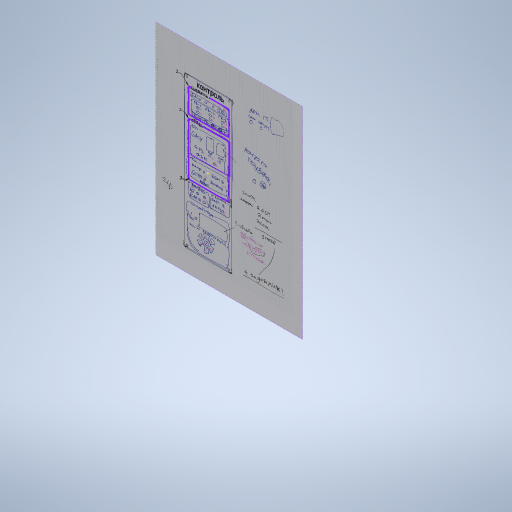
# Autodesk Inventor part: блок контроля
Saved by Autodesk Inventor 2023.1 (Build 271208000, 208)
## iProperties
Created: 2023-02-23
Part Number: блок контроля
Material: Типовые
Document SubType Name: Modeling
Designer: User
Density: 1 g/cm^3
Appearance: По умолчанию
Author: User
Autodesk Inventor part; units mm, degrees
ref_plane "YZ Plane" through (0, 0, 0) normal (1, 0, 0) x (0, 1, 0)
ref_plane "XZ Plane" through (0, 0, 0) normal (0, 1, 0) x (-1, 0, 0)
ref_plane "XY Plane" through (0, 0, 0) normal (0, 0, 1) x (1, 0, 0)
sketch "Эскиз1" plane through (0, 0, 0) normal (0, 0, 1) x (1, 0, 0)
  line L0 (-35, 111.5) -> (35, 111.5)
  line L1 (35, 111.5) -> (35, -111.5)
  line L2 (35, -111.5) -> (-35, -111.5)
  line L3 (-35, -111.5) -> (-35, 111.5)
  line L4 (0, -156.1) -> (0, 156.1) projected
  line L5 (-49, 0) -> (49, 0) projected
  line L6 (-30, 106.5) -> (30, 106.5)
  line L7 (30, 106.5) -> (30, -106.5)
  line L8 (30, -106.5) -> (-30, -106.5)
  line L9 (-30, -106.5) -> (-30, 106.5)
  circle A0 centre (-31, 107.5) radius 1.5
  circle A1 centre (-31, 107.5) radius 3.5
  circle A2 centre (31, 107.5) radius 1.5
  circle A3 centre (31, 107.5) radius 3.5
  circle A4 centre (-31, -107.5) radius 1.5
  circle A5 centre (-31, -107.5) radius 3.5
  circle A6 centre (31, -107.5) radius 1.5
  circle A7 centre (31, -107.5) radius 3.5
  point P0 (0, 0)
  dimension "d0" = 70
  dimension "d1" = 223
  dimension "d2" = 5
  dimension "d3" = 5
  dimension "d4" = 5
  dimension "d5" = 5
  dimension "d6" = 3
  dimension "d7" = 7
  dimension "d8" = 3
  dimension "d9" = 7
  dimension "d10" = 3
  dimension "d11" = 7
  dimension "d12" = 3
  dimension "d13" = 7
  dimension "d14" = 1
  dimension "d15" = 1
  dimension "d16" = 1
  dimension "d17" = 1
  dimension "d18" = 1
  dimension "d19" = 1
  dimension "d20" = 1
  dimension "d21" = 1
  constraints: 16 end point, 8 centre point, 4 coincident, 4 parallel, 2 horizontal, 2 perpendicular, 2 other
  measures "d0" distance between parallel lines of L1 L3
  measures "d1" distance between parallel lines of L2 L0
  measures "d2" distance between parallel lines of L6 L0
  measures "d3" distance between parallel lines of L1 L7
  measures "d4" distance between parallel lines of L3 L9
  measures "d5" distance between parallel lines of L2 L8
  measures "d6" diameter of A0
  measures "d7" diameter of A1
  measures "d8" diameter of A2
  measures "d9" diameter of A3
  measures "d10" diameter of A4
  measures "d11" diameter of A5
  measures "d12" diameter of A6
  measures "d13" diameter of A7
  measures "d14" distance from line of L9 A0.centre
  measures "d15" distance from line of A0.centre L6
  measures "d16" distance from line of L8 A4.centre
  measures "d17" distance from line of L9 A4.centre
  measures "d18" distance from line of L8 A6.centre
  measures "d19" distance from line of A7.centre L7
  measures "d20" distance from line of L6 A2.centre
  measures "d21" distance from line of L7 A2.centre
extrude "Выдавливание1" add sketch "Эскиз1" along normal blind 2 contours L0 L4 L6 A1 L9 L5 L3 | L0 L1 L5 L7 A3 L6 L4 | L5 L9 A5 L8 L4 L2 L3 | L6 A3 L7 L5 L4 | L4 L5 L9 A1 L6 | L5 L4 L8 A5 L9 | L1 L2 L4 L8 A7 L7 L5 | L5 L7 A7 L8 L4 | A1 L9 A0 L6 | L6 A0 L9 A1 | A3 L7 A2 L6 | L6 A2 L7 A3 | A5 L8 A4 L9 | L9 A4 L8 A5 | A7 L8 A6 L7 | L7 A6 L8 A7
fillet "Сопряжение1" radius 3 4 edges at (-35, -111.5, 1) (-35, 111.5, 1) (35, 111.5, 1) (35, -111.5, 1)
sketch "Эскиз2" plane through (0, 0, 2) normal (0, 0, 1) x (1, 0, 0)
  line L0 (-76.7343, 154.5381) -> (139.2503, 154.5381) construction
  line L1 (139.2503, 154.5381) -> (139.2503, -142.4726) construction
  line L2 (139.2503, -142.4726) -> (-76.7343, -142.4726) construction
  line L3 (-76.7343, -142.4726) -> (-76.7343, 154.5381) construction
  line L4 (-16.9113, 107.032) -> (17.9169, 107.032) construction
  line L5 (17.9169, 107.032) -> (17.9169, 100.7451) construction
  line L6 (17.9169, 100.7451) -> (-16.9113, 100.7451) construction
  line L7 (-16.9113, 100.7451) -> (-16.9113, 107.032) construction
  line L8 (31.258, 95.6248) -> (31.258, 62.5304)
  line L9 (29.258, 60.5304) -> (-27.4022, 60.5304)
  line L10 (-29.4022, 62.5304) -> (-29.4022, 95.6248)
  arc A0 (-27.4022, 97.6248) -> (-29.4022, 95.6248) centre (-27.4022, 95.6248) ccw
  arc A1 (31.258, 95.6248) -> (29.258, 97.6248) centre (29.258, 95.6248) ccw
  arc A2 (29.258, 60.5304) -> (31.258, 62.5304) centre (29.258, 62.5304) ccw
  arc A3 (-29.4022, 62.5304) -> (-27.4022, 60.5304) centre (-27.4022, 62.5304) ccw
  arc A4 (-27.4022, 96.6248) -> (-28.4022, 95.6248) centre (-27.4022, 95.6248) ccw
  line L11 (-28.4022, 95.6248) -> (-28.4022, 62.5304)
  arc A5 (-28.4022, 62.5304) -> (-27.4022, 61.5304) centre (-27.4022, 62.5304) ccw
  line L12 (-27.4022, 61.5304) -> (29.258, 61.5304)
  arc A6 (29.258, 61.5304) -> (30.258, 62.5304) centre (29.258, 62.5304) ccw
  line L13 (30.258, 62.5304) -> (30.258, 95.6248)
  arc A7 (30.258, 95.6248) -> (29.258, 96.6248) centre (29.258, 95.6248) ccw
  line L14 (-25.7338, 97.6248) -> (-25.7338, 96.6248)
  line L15 (-24.8875, 98.8096) -> (-4.5511, 98.8096) construction
  line L16 (-4.5511, 98.8096) -> (-4.5511, 95.9853) construction
  line L17 (-4.5511, 95.9853) -> (-24.8875, 95.9853) construction
  line L18 (-24.8875, 95.9853) -> (-24.8875, 98.8096) construction
  line L19 (1.4856, 96.6248) -> (1.4856, 97.6248)
  line L20 (-27.4022, 97.6248) -> (-25.7338, 97.6248)
  line L21 (1.4856, 97.6248) -> (29.258, 97.6248)
  line L22 (29.258, 96.6248) -> (1.4856, 96.6248)
  line L23 (-25.7338, 96.6248) -> (-27.4022, 96.6248)
  line L24 (31.258, 54.2392) -> (31.258, 12.1954)
  line L25 (-29.4022, 12.1954) -> (-29.4022, 54.2392)
  arc A8 (-27.4022, 56.2392) -> (-29.4022, 54.2392) centre (-27.4022, 54.2392) ccw
  arc A9 (31.258, 54.2392) -> (29.258, 56.2392) centre (29.258, 54.2392) ccw
  arc A10 (-27.4022, 55.2392) -> (-28.4022, 54.2392) centre (-27.4022, 54.2392) ccw
  line L26 (-28.4022, 54.2392) -> (-28.4022, 12.1954)
  line L27 (30.258, 12.1954) -> (30.258, 54.2392)
  arc A11 (30.258, 54.2392) -> (29.258, 55.2392) centre (29.258, 54.2392) ccw
  line L28 (-25.7338, 56.2392) -> (-25.7338, 55.2392)
  line L29 (-24.6363, 58.99) -> (-4.7949, 58.99) construction
  line L30 (-4.7949, 58.99) -> (-4.7949, 51.439) construction
  line L31 (-4.7949, 51.439) -> (-24.6363, 51.439) construction
  line L32 (-24.6363, 51.439) -> (-24.6363, 58.99) construction
  line L33 (31.258, 12.1954) -> (31.258, -20.0847)
  line L34 (29.258, -22.0847) -> (-27.4022, -22.0847)
  line L35 (-29.4022, -20.0847) -> (-29.4022, 12.1954)
  line L36 (29.9651, 12.1954) -> (29.9651, -20.0847)
  line L37 (28.9651, -21.0847) -> (-27.4022, -21.0847)
  line L38 (-28.4022, -20.0847) -> (-28.4022, 12.1954)
  arc A12 (-29.4022, -20.0847) -> (-27.4022, -22.0847) centre (-27.4022, -20.0847) ccw
  arc A13 (29.258, -22.0847) -> (31.258, -20.0847) centre (29.258, -20.0847) ccw
  arc A14 (-28.4022, -20.0847) -> (-27.4022, -21.0847) centre (-27.4022, -20.0847) ccw
  arc A15 (28.9651, -21.0847) -> (29.9651, -20.0847) centre (28.9651, -20.0847) ccw
  line L39 (-7.2077, 56.2392) -> (-7.2077, 55.2392)
  line L40 (-27.4022, 56.2392) -> (-24.6363, 56.2392)
  line L41 (-7.2077, 56.2392) -> (29.258, 56.2392)
  line L42 (29.258, 55.2392) -> (-7.2077, 55.2392)
  line L43 (-24.6363, 55.2392) -> (-27.4022, 55.2392)
  point P0 (0, 0)
  dimension "d28" = 2
  dimension "d32" = 2
  dimension "d38" = 1
  dimension "d39" = 2
  dimension "d40" = 1
  constraints: 56 end point, 32 point on circle, 24 tangent, 16 centre point, 16 perpendicular, 10 parallel, 6 equal radius, 4 horizontal, 4 point on line, 1 vertical alignment, 16 other
  measures "d28" radius of A0
  measures "d32" radius of A8
  measures "d38" distance between parallel lines of L37 L34
  measures "d39" radius of A12
  measures "d40" radius of A14
sketch "Эскиз3" plane through (0, 0, 2) normal (0, 0, 1) x (1, 0, 0)
  line L0 (-29.1336, 55.9595) -> (31.8891, 55.9595)
  line L1 (31.8891, 55.9595) -> (31.8891, 11.7105)
  line L2 (31.8891, 11.7105) -> (-29.1336, 11.7105)
  line L3 (-29.1336, 11.7105) -> (-29.1336, 55.9595)
  point P0 (0, 0)
  constraints: 8 end point, 2 parallel, 1 horizontal, 1 perpendicular
